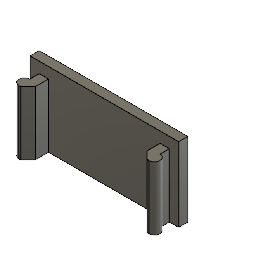
PSRSoundMeter (Autodesk Fusion 360 archive; units mm, degrees)
design "End Cap"
Autodesk Fusion 360 part; units mm, degrees
note: some values were not read from the file. Set by a fixed rule: which face or edge a step refers to.
sketch "Sketch1" plane through (0, 0, 0) normal (0, 0, 1) x (1, 0, 0)
  line L0 (-25.4, 12.7) -> (25.4, 12.7)
  line L1 (25.4, 12.7) -> (25.4, -12.7)
  line L2 (25.4, -12.7) -> (-25.4, -12.7)
  line L3 (-25.4, -12.7) -> (-25.4, 12.7)
  line L4 (-25.4, 12.7) -> (25.4, -12.7) construction
  dimension "d1" = 50.8
  dimension "d2" = 25.4
  constraint horizontal L0
  constraint vertical L1
  constraint horizontal L2
  constraint vertical L3
  constraint midpoint origin L4
  measures "d1" distance of L0.start L0.end
  measures "d2" distance of L0.end L1.end
extrude "Extrude1" add sketch "Sketch1" along normal mid plane 3.175
sketch "Sketch2" plane through (0, 0, 1.5875) normal (0, 0, 1) x (1, 0, 0)
  line L0 (-25.4, -12.7) -> (25.4, -12.7)
  line L1 (25.4, -12.7) -> (25.4, 12.7)
  line L2 (25.4, 12.7) -> (-25.4, 12.7)
  line L3 (-25.4, 12.7) -> (-25.4, -12.7)
  line L4 (-22.225, 9.025) -> (-19.05, 9.025)
  line L5 (-19.05, 9.025) -> (-19.05, -12.7)
  line L6 (-19.05, -12.7) -> (-22.225, -12.7)
  line L7 (-22.225, -12.7) -> (-22.225, 9.025)
  dimension "d5" = 3.175
  dimension "d6" = 3.675
  dimension "d15" = 3.175
  constraint horizontal L4
  constraint vertical L5
  constraint horizontal L6
  constraint vertical L7
  constraint coincident L0 L5.end
  measures "d5" distance of L4.start L4.end
  measures "d6" distance of L2 L4
  measures "d15" distance of L3 L7
extrude "Extrude2" add sketch "Sketch2" along normal blind 6.985 contours L0 L4 L5 L6 L7
sketch "Sketch3" plane through (0, -12.7, 0) normal (0, -1, 0) x (1, 0, 0)
  line L0 (-22.225, 1.5875) -> (-19.05, 1.5875)
  line L1 (-19.05, 1.5875) -> (-19.05, 8.5725)
  line L2 (-19.05, 8.5725) -> (-22.225, 8.5725)
  line L3 (-22.225, 8.5725) -> (-22.225, 1.5875)
  line L4 (-22.225, 8.5725) -> (-22.225, 4.7625)
  arc A0 (-22.225, 8.5725) -> (-22.225, 4.7625) centre (-22.225, 6.6675) ccw
  dimension "d16" = 1.905
  constraint coincident L2.end L3.start
  constraint coincident L3 L4.end
  constraint perpendicular L2 L4
  constraint tangent L2 A0
  measures "d16" radius of A0
extrude "Extrude3" add sketch "Sketch3" against normal up to surface (21.725 mm away)
chamfer "Chamfer1" distance 2.54 angle 45 1 edges at (-19.05, -1.8375, 8.5725)
mirror "Mirror1" about plane through (0, 0, 0) normal (1, 0, 0) of "Extrude2", "Extrude3", "Chamfer1"
sketch "Sketch4" plane through (0, 0, -1.5875) normal (0, 0, -1) x (-1, 0, 0)
  line L0 (-25.4, -12.7) -> (25.4, -12.7)
  line L1 (25.4, -12.7) -> (25.4, 12.7)
  line L2 (25.4, 12.7) -> (-25.4, 12.7)
  line L3 (-25.4, 12.7) -> (-25.4, -12.7)
  line L4 (-10, -7.7) -> (10, -7.7)
  line L5 (10, -7.7) -> (10, -12.7)
  line L6 (10, -12.7) -> (-10, -12.7)
  line L7 (-10, -12.7) -> (-10, -7.7)
  dimension "d17" = 20
  dimension "d18" = 5
  constraint horizontal L4
  constraint vertical L5
  constraint horizontal L6
  constraint vertical L7
  constraint midpoint L0 L6
  measures "d17" distance of L4.start L4.end
  measures "d18" distance of L4.end L5.end
extrude "Extrude4" add sketch "Sketch4" along normal blind 20 contours L0 L4 L5 L6 L7
fillet "Fillet1" radius 7 1 edges at (0, -7.7, -1.5875)
sketch "Sketch5" plane through (0, -7.7, 0) normal (0, 1, 0) x (-1, 0, 0)
  line L0 (10, -8.5875) -> (-10, -8.5875)
  line L1 (-10, -8.5875) -> (-10, -21.5875)
  line L2 (-10, -21.5875) -> (10, -21.5875)
  line L3 (10, -21.5875) -> (10, -8.5875)
  circle A0 centre (0, -11.5875) radius 10
  circle A1 centre (0, -14.5875) radius 2.286
  line L4 (0, -14.5875) -> (0, -11.5875) construction
  dimension "d23" = 4.572
  dimension "d24" = 3
  constraint tangent L3 A0
  constraint tangent L2 A0
  constraint tangent L1 A0
  constraint coincident A1.centre L4.start
  constraint coincident A0.centre L4.end
  constraint vertical L4
  measures "d23" diameter of A1
  measures "d24" distance of A1.centre A0.centre
extrude "Extrude5" cut sketch "Sketch5" against normal up to surface (5 mm away) contours L2 L3 A0 | L1 L2 A0 | A1
chamfer "Chamfer2" distance 2 angle 45 1 edges at (2.1313, -7.7, -13.7608)
equation "d6 = 0.125 in + 0.5 mm"
equation "d16 = ( 0.15 / 2 ) * 1 in"

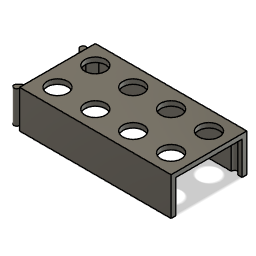
design "Modular+LED+Bar"
Autodesk Fusion 360 part; units mm, degrees
sketch "Sketch1" plane through (0, 0, 0) normal (1, 0, 0) x (0, 0, -1)
  line L0 (-25.4, 12.7) -> (25.4, 12.7)
  line L1 (25.4, 12.7) -> (25.4, -12.7)
  line L2 (25.4, -12.7) -> (-25.4, -12.7)
  line L3 (-25.4, -12.7) -> (-25.4, 12.7)
  line L4 (-25.4, 12.7) -> (25.4, -12.7) construction
  line L5 (25.4, 12.7) -> (-25.4, -12.7) construction
  dimension "d1" = 50.8
  dimension "d43" = 25.4
  constraint horizontal L0
  constraint perpendicular L0 L1
  constraint parallel L0 L2
  constraint parallel L1 L3
  constraint coincident L4 origin
  constraint coincident L5 origin
  measures "d1" distance of L0.start L0.end
  measures "d43" distance of L0.end L1.end
extrude "Extrude1" add sketch "Sketch1" along normal mid plane 101.6 makes body 1
shell "Shell1" thickness 3.175 removed faces 3 at (-50.8, 4.2333, 8.4667) at (16.9333, -12.7, -8.4667) at (50.8, 4.2333, 8.4667) on bodies 1
hole "Hole1" at (-38.1, 12.7, -12.7) direction (0, -1, 0) diameter 13.85 end through all bodies 1
pattern_linear "R-Pattern1" count 4 spacing 25.4 along (1, 0, 0) of "Hole1"
sketch "Sketch2" plane through (-50.8, 0, 0) normal (-1, 0, 0) x (0, 0, 1)
  line L0 (-22.225, -12.7) -> (-22.225, 9.525)
  line L1 (-22.225, 9.525) -> (22.225, 9.525)
  line L2 (22.225, 9.525) -> (22.225, -12.7)
  line L3 (22.225, -12.7) -> (25.4, -12.7)
  line L4 (25.4, -12.7) -> (25.4, 12.7)
  line L5 (25.4, 12.7) -> (-25.4, 12.7)
  line L6 (-25.4, 12.7) -> (-25.4, -12.7)
  line L7 (-25.4, -12.7) -> (-22.225, -12.7)
  line L8 (-22.225, 9.525) -> (-19.05, 9.525)
  line L9 (-19.05, 9.525) -> (-19.05, -12.7)
  line L10 (-19.05, -12.7) -> (-22.225, -12.7)
  line L11 (-22.225, -12.7) -> (-22.225, 9.525)
  constraint horizontal L8
  constraint vertical L9
  constraint horizontal L10
  constraint vertical L11
  constraint coincident L0.end L1.start
  constraint collinear L7 L10
  constraint equal L7 L10
extrude "Extrude2" add sketch "Sketch2" along normal blind 6.985 separate body contours L0 L1 L8 L9 L10 L11 makes body 2
sketch "Sketch3" plane through (0, -12.7, 0) normal (0, -1, 0) x (1, 0, 0)
  line L0 (-50.8, -22.225) -> (-50.8, -19.05)
  line L1 (-50.8, -19.05) -> (-57.785, -19.05)
  line L2 (-57.785, -19.05) -> (-57.785, -22.225)
  line L3 (-57.785, -22.225) -> (-50.8, -22.225)
  line L4 (-50.8, -19.05) -> (-45.3007, -22.225)
  line L5 (-45.3007, -22.225) -> (-50.8, -22.225)
  line L6 (50.8, -22.225) -> (-50.8, -22.225)
  dimension "d15" = 30
  constraint coincident L0.end L1.start
  constraint coincident L0 L3.end
  constraint perpendicular L0 L5
  constraint collinear L5 L6
  measures "d15" angle of L4 L5
extrude "Extrude3" add sketch "Sketch3" against normal up to surface (22.225 mm away) contours L0 L4 L5 L6 bodies 1 2
sketch "Sketch4" plane through (0, -12.7, 0) normal (0, -1, 0) x (1, 0, 0)
  line L0 (-50.8, -19.05) -> (-57.785, -19.05)
  line L1 (-57.785, -19.05) -> (-57.785, -22.225)
  line L2 (-57.785, -22.225) -> (-50.8, -22.225)
  line L3 (-50.8, -22.225) -> (-50.8, -25.4)
  line L4 (-50.8, -25.4) -> (50.8, -25.4)
  line L5 (50.8, -25.4) -> (50.8, -22.225)
  line L6 (50.8, -22.225) -> (-45.3007, -22.225)
  line L7 (-45.3007, -22.225) -> (-50.8, -19.05)
  line L8 (-57.785, -22.225) -> (-53.975, -22.225)
  arc A0 (-57.785, -22.225) -> (-53.975, -22.225) centre (-55.88, -22.225) ccw
  dimension "d18" = 3.81
  constraint coincident L1.end L2.start
  constraint coincident L2 L8.end
  constraint perpendicular L1 L8
  constraint tangent L1 A0
  measures "d18" distance of L1.end L8.end
extrude "Extrude4" add sketch "Sketch4" against normal up to surface (21.725 mm away) contours L2 L8 A0 bodies 1
sketch "Sketch5" plane through (0, -12.7, 0) normal (0, -1, 0) x (1, 0, 0)
  line L0 (-50.8, -19.05) -> (-57.785, -19.05)
  line L1 (-57.785, -19.05) -> (-57.785, -22.225)
  arc A0 (-57.785, -22.225) -> (-53.975, -22.225) centre (-55.88, -22.225) ccw
  line L2 (-53.975, -22.225) -> (-50.8, -22.225)
  line L3 (-50.8, -22.225) -> (-50.8, -25.4)
  line L4 (-50.8, -25.4) -> (50.8, -25.4)
  line L5 (50.8, -25.4) -> (50.8, -22.225)
  line L6 (50.8, -22.225) -> (-45.3007, -22.225)
  line L7 (-45.3007, -22.225) -> (-50.8, -19.05)
  line L8 (47.9425, -22.225) -> (43.4975, -22.225)
  arc A1 (43.4975, -22.225) -> (47.9425, -22.225) centre (45.72, -22.2063) ccw
  line L9 (47.9425, -22.225) -> (43.4975, -22.225)
  arc A2 (43.4975, -22.225) -> (47.9425, -22.225) centre (45.72, -22.2063) ccw
  dimension "d21" = 4.445
  dimension "d42" = 5.08
  dimension "d44" = 4.445
  constraint coincident L6 L8.start
  constraint coincident L6 L8.end
  measures "d21" distance of L8.start L8.end
  measures "d42" distance of L5 A1.centre
  measures "d44" distance of L8.end L8.start
extrude "Extrude5" cut sketch "Sketch5" against normal up to surface (22.225 mm away) contours L6 L8 A1 L9 A2 bodies 1
chamfer "Chamfer1" distance 2.54 angle 45 1 edges at (-57.785, -1.5875, -19.05) on bodies 1
sketch "Sketch8" plane through (0, 0, -22.225) normal (0, 0, -1) x (-1, 0, 0)
  line L0 (53.975, 9.025) -> (57.785, 9.025)
  line L1 (57.785, 9.025) -> (57.785, 9.525)
  line L2 (57.785, 9.525) -> (50.8, 9.525)
  line L3 (50.8, 9.525) -> (50.8, -12.7)
  line L4 (50.8, -12.7) -> (53.975, -12.7)
  line L5 (53.975, -12.7) -> (53.975, 9.025)
  line L6 (50.8, 9.525) -> (57.785, 9.525)
  line L7 (57.785, 9.525) -> (57.785, 9.025)
  line L8 (57.785, 9.025) -> (50.8, 9.025)
  line L9 (50.8, 9.025) -> (50.8, 9.525)
  constraint horizontal L6
  constraint vertical L7
  constraint horizontal L8
  constraint vertical L9
  constraint coincident L0.end L1.start
  constraint coincident L2.end L3.start
extrude "Extrude8" cut sketch "Sketch8" against normal up to surface (3.175 mm away) contours L0 L1 L2 L3 L6 L7 L8 L9 bodies 1
mirror "Mirror1" about plane through (0, 0, 0) normal (0, 0, 1) of "Hole1", "R-Pattern1", "Extrude2", "Extrude3", "Extrude4", "Extrude5", "Chamfer1", "Extrude8"
